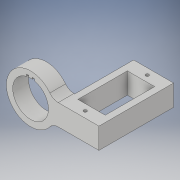
# Autodesk Inventor part: servo mount
Saved by Autodesk Inventor 2019.3 (Build 233278000, 278)
## iProperties
Created: 2019-04-01
Part Number: servo mount
Material: Generic
Document SubType Name: Modeling
Designer: peter
Density: 1 g/cm^3
Appearance: Default
Author: peter
Autodesk Inventor part; units mm, degrees
ref_plane "YZ Plane" through (0, 0, 0) normal (1, 0, 0) x (0, 1, 0)
ref_plane "XZ Plane" through (0, 0, 0) normal (0, 1, 0) x (-1, 0, 0)
ref_plane "XY Plane" through (0, 0, 0) normal (0, 0, 1) x (1, 0, 0)
sketch "Sketch1" plane through (0, 0, 0) normal (0, 1, 0) x (-1, 0, 0)
  line L0 (0, 0) -> (13, 0)
  line L1 (13, 0) -> (13, -23.5)
  line L2 (13, -23.5) -> (0, -23.5)
  line L3 (0, -23.5) -> (0, 0)
  line L4 (0, 0) -> (-3, 0) construction
  line L5 (-3, 0) -> (-3, 6) construction
  line L6 (-3, 6) -> (0, 6) construction
  line L7 (0, 6) -> (0, 0) construction
  line L8 (-3, 6) -> (16, 6)
  line L9 (16, 6) -> (16, -29.5)
  line L10 (16, -29.5) -> (-3, -29.5)
  line L11 (-3, -29.5) -> (-3, 6)
  line L12 (6.5, 6) -> (6.5, 3) construction
  circle A0 centre (6.5, 3) radius 0.75
  line L13 (16, -11.75) -> (-3, -11.75) construction
  circle A1 centre (6.5, -26.5) radius 0.75
  dimension "d6" = 13
  dimension "d7" = 23.5
  dimension "d8" = 3
  dimension "d9" = 6
  dimension "d10" = 19
  dimension "d11" = 35.5
  dimension "d14" = 3
  dimension "d15" = 1.5
  constraints: 28 end point, 6 parallel, 3 horizontal, 3 midpoint, 3 perpendicular, 2 centre point, 1 coincident, 1 symmetric about line, 1 vertical, 1 other
  measures "d6" distance of L1.end L2.end
  measures "d7" distance of L0.end L1.end
  measures "d8" distance of L5.end L6.end
  measures "d9" distance of L4.end L5.end
  measures "d10" distance of L9.end L10.end
  measures "d11" distance of L8.end L9.end
  measures "d14" distance of L12.start L12.end
  measures "d15" diameter of A0
extrude "Extrusion1" add sketch "Sketch1" along normal blind 10
sketch "Sketch2" plane through (-16, 0, 6) normal (0, 0, 1) x (1, 0, 0)
  line L0 (0, 0) -> (0, 10) construction
  line L1 (-5, 5) -> (-13.5, 5) construction
  line L2 (19, 0) -> (0, 0) projected
  line L3 (19, 0) -> (19, 10) projected
  line L4 (0, 10) -> (19, 10) projected
  line L5 (0, 0) -> (0, 10) projected
  arc A0 (-4.3527, 11.9697) -> (-4.3527, -1.9697) centre (-13.5, 5) ccw
  line L6 (-13.5, 5) -> (-13.5, 13.5) construction
  line L7 (-13.5, 5) -> (-12.7, 5) construction
  line L8 (-12.7, 5) -> (-11.5, 5) construction
  line L9 (-12.7, 5) -> (-12.7, 14.2655) construction
  line L10 (-11.5, 5) -> (-11.5, 14.0824) construction
  line L11 (-11.5, 13.2614) -> (-11.5, 14.0824)
  line L12 (-12.7, 13.4623) -> (-12.7, 14.2655)
  arc A1 (-11.5, 14.0824) -> (-12.7, 14.2655) centre (-13.5, 5) ccw
  arc A2 (-5, 1.2264) -> (-5, 8.7736) centre (-13.5, 5) ccw construction
  line L13 (-15.5, 13.2614) -> (-15.5, 14.0824)
  line L14 (-14.3, 13.4623) -> (-14.3, 14.2655)
  arc A3 (-14.3, 14.2655) -> (-15.5, 14.0824) centre (-13.5, 5) ccw
  arc A4 (-12.7, 13.4623) -> (-14.3, 13.4623) centre (-13.5, 5) ccw
  arc A5 (-15.5, 13.2614) -> (-11.5, 13.2614) centre (-13.5, 5) ccw
  line L15 (0, 10) -> (19, 10) construction
  line L16 (0, 10) -> (-0.3756, 10)
  line L17 (0, 0) -> (-0.3756, 0)
  arc A6 (-4.3527, 11.9697) -> (-0.3756, 10) centre (-0.3756, 15) ccw
  arc A7 (-0.3756, 0) -> (-4.3527, -1.9697) centre (-0.3756, -5) ccw
  line L18 (0, 10) -> (0, 0)
  point P0 (16, 0)
  point P1 (-3.1438, 10)
  dimension "d16" = 8.5
  dimension "d18" = 23
  dimension "d19" = 0.8
  dimension "d20" = 1.2
  dimension "d25" = 5
  constraints: 26 end point, 18 point on circle, 8 centre point, 5 point on line, 4 symmetric about line, 4 tangent, 3 coincident, 3 parallel, 2 collinear, 1 equal radius, 1 horizontal, 1 perpendicular, 1 vertical, 1 other
  measures "d16" distance of L1.start L1.end
  measures "d18" diameter of A0
  measures "d19" distance of L6.start L7.end
  measures "d20" distance of L7.end L8.end
  measures "d25" radius of A6
extrude "Extrusion2" add sketch "Sketch2" against normal blind 7.5 contours L17 A7 A0 A6 L16 L5
body "Solid1"
